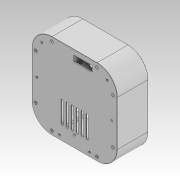
# Autodesk Inventor part: J1_Base
Saved by Autodesk Inventor 2020 (Build 240168000, 168)
## iProperties
Created: 2021-03-23
Part Number: J1_Base
Material: Generic
Document SubType Name: Modeling
Designer: DDeGo
Density: 1 g/cm^3
Appearance: Default
Author: DDeGo
Autodesk Inventor part; units mm, degrees
sketch "Block1" plane through (0, 0, 0) normal (0, 0, 1) x (1, 0, 0)
  circle A0 centre (112.1187, 97.7562) radius 2.75
  line L0 (90.8687, 90.2562) -> (90.8687, 49.9679) construction
  circle A1 centre (83.3687, 50.2562) radius 2.75
  line L1 (75.8687, 49.9679) -> (75.8687, 122.7562) construction
  line L2 (75.8687, 49.9679) -> (90.8687, 49.9679) construction
  circle A2 centre (83.3687, 115.2562) radius 2.75
  line L3 (90.8687, 90.2562) -> (190.8687, 90.2562) construction
  line L4 (75.8687, 122.7562) -> (205.8687, 122.7562) construction
  circle A3 centre (140.8687, 115.2562) radius 2.75
  circle A4 centre (169.6187, 97.7562) radius 2.75
  circle A5 centre (198.3687, 115.2562) radius 2.75
  line L5 (190.8687, 90.2562) -> (190.8687, 40.2562) construction
  line L6 (205.8687, 40.2562) -> (205.8687, 122.7562) construction
  circle A6 centre (198.3687, 50.2562) radius 2.75
  line L7 (205.8687, 40.2562) -> (190.8687, 40.2562) construction
  line L8 (83.3687, 115.2562) -> (140.8687, 115.2562) construction
  line L9 (140.8687, 115.2562) -> (198.3687, 115.2562) construction
  line L10 (198.3687, 115.2562) -> (198.3687, 50.2562) construction
  line L11 (198.3687, 50.2562) -> (83.3687, 50.2562) construction
  line L12 (83.3687, 50.2562) -> (83.3687, 115.2562) construction
  line L13 (112.1187, 115.2562) -> (112.1187, 97.7562) construction
  line L14 (169.6187, 115.2562) -> (169.6187, 97.7562) construction
  line L15 (169.6187, 97.7562) -> (112.1187, 97.7562) construction
  point P0 (142.3997, 87.8737)
  point P1 (140.8687, 90.2562)
  point P2 (140.8687, 90.2562)
  dimension "d9" = 5.5
  dimension "d10" = 57.5
  dimension "d11" = 7.5
  dimension "d12" = 7.5
  dimension "d13" = 7.5
  dimension "d14" = 17.5
  dimension "d15" = 7.5
  dimension "d16" = 10
  dimension "d17" = 65
  dimension "d18" = 7.5
  dimension "d19" = 7.5
  measures "d9" diameter of A0
  measures "d10" distance of L8.start L8.end
  measures "d11" distance between parallel lines of L6 L10
  measures "d12" distance between parallel lines of L4 L9
  measures "d13" distance between parallel lines of L1 L12
  measures "d14" distance of L13.start L13.end
  measures "d15" distance between parallel lines of L3 L15
  measures "d16" distance between parallel lines of L7 L11
  measures "d17" distance of L9.end L10.end
  measures "d18" distance from line of L5 L10.end
  measures "d19" distance between parallel lines of L12 L0
sketch "Sketch1" plane through (0, 0, 0) normal (0, 0, 1) x (1, 0, 0)
  line L0 (45, -85) -> (-45, -85)
  line L1 (-85, -45) -> (-85, 45)
  line L2 (-45, 85) -> (45, 85)
  line L3 (85, 45) -> (85, -45)
  line L4 (85, -85) -> (-85, 85) construction
  line L5 (-85, -85) -> (85, 85) construction
  arc A0 (-45, 85) -> (-85, 45) centre (-45, 45) ccw
  arc A1 (85, 45) -> (45, 85) centre (45, 45) ccw
  arc A2 (45, -85) -> (85, -45) centre (45, -45) ccw
  arc A3 (-85, -45) -> (-45, -85) centre (-45, -45) ccw
  point P0 (0, 0)
  dimension "d1" = 170
  dimension "d2" = 170
  dimension "d3" = 40
  constraints: 12 end point, 8 point on circle, 8 point on line, 8 tangent, 4 centre point, 3 equal radius, 2 midpoint, 2 parallel, 1 horizontal, 1 perpendicular
  measures "d1" distance between parallel lines of L3 L1
  measures "d2" distance between parallel lines of L0 L2
  measures "d3" radius of A0
extrude "Extrusion1" add sketch "Sketch1" along normal blind 62
sketch "Sketch2" plane through (0, 0, 62) normal (0, 0, 1) x (1, 0, 0)
  line L0 (0, 0) -> (-85, 0) construction
  line L1 (-85, 45) -> (-85, -45) projected
  line L2 (0, 0) -> (0, 52.5) construction
  line L3 (45, 85) -> (-45, 85) projected
  circle A0 centre (-28.75, 60) radius 2.75
  line L4 (-50, 52.5) -> (-50, 12.2116) construction
  circle A1 centre (-57.5, 12.5) radius 2.75
  line L5 (-65, 12.2116) -> (-65, 85) construction
  line L6 (-65, 12.2116) -> (-50, 12.2116) construction
  circle A2 centre (-57.5, 77.5) radius 2.75
  line L7 (-50, 52.5) -> (50, 52.5) construction
  line L8 (-65, 85) -> (65, 85) construction
  circle A3 centre (0, 77.5) radius 2.75
  circle A4 centre (28.75, 60) radius 2.75
  circle A5 centre (57.5, 77.5) radius 2.75
  line L9 (50, 52.5) -> (50, 2.5) construction
  line L10 (65, 2.5) -> (65, 85) construction
  circle A6 centre (57.5, 12.5) radius 2.75
  line L11 (65, 2.5) -> (50, 2.5) construction
  line L12 (-57.5, 77.5) -> (0, 77.5) construction
  line L13 (0, 77.5) -> (57.5, 77.5) construction
  line L14 (57.5, 77.5) -> (57.5, 12.5) construction
  line L15 (57.5, 12.5) -> (-57.5, 12.5) construction
  line L16 (-57.5, 12.5) -> (-57.5, 77.5) construction
  line L17 (-28.75, 77.5) -> (-28.75, 60) construction
  line L18 (28.75, 77.5) -> (28.75, 60) construction
  line L19 (28.75, 60) -> (-28.75, 60) construction
  circle A7 centre (-28.75, -60) radius 2.75
  line L20 (-50, -52.5) -> (-50, -12.2116) construction
  circle A8 centre (-57.5, -12.5) radius 2.75
  line L21 (-65, -12.2116) -> (-65, -85) construction
  line L22 (-65, -12.2116) -> (-50, -12.2116) construction
  circle A9 centre (-57.5, -77.5) radius 2.75
  line L23 (-50, -52.5) -> (50, -52.5) construction
  line L24 (-65, -85) -> (65, -85) construction
  circle A10 centre (0, -77.5) radius 2.75
  circle A11 centre (28.75, -60) radius 2.75
  circle A12 centre (57.5, -77.5) radius 2.75
  line L25 (50, -52.5) -> (50, -2.5) construction
  line L26 (65, -2.5) -> (65, -85) construction
  circle A13 centre (57.5, -12.5) radius 2.75
  line L27 (65, -2.5) -> (50, -2.5) construction
  line L28 (-57.5, -77.5) -> (0, -77.5) construction
  line L29 (0, -77.5) -> (57.5, -77.5) construction
  line L30 (57.5, -77.5) -> (57.5, -12.5) construction
  line L31 (57.5, -12.5) -> (-57.5, -12.5) construction
  line L32 (-57.5, -12.5) -> (-57.5, -77.5) construction
  line L33 (-28.75, -77.5) -> (-28.75, -60) construction
  line L34 (28.75, -77.5) -> (28.75, -60) construction
  line L35 (28.75, -60) -> (-28.75, -60) construction
  constraints: 4 end point, 2 horizontal, 1 midpoint, 1 vertical, 2 other
extrude "Extrusion2" [suppressed]
ref_plane "Work Plane1" through (0, 0, -15) normal (0, 0, -1) x (-1, 0, 0)
sketch "Sketch3" plane through (0, 0, -15) normal (0, 0, -1) x (-1, 0, 0)
  circle A0 centre (0, 0) radius 87.5
  line L0 (-85, -45) -> (-85, 45) construction
  dimension "d27" = 175
  constraints: 1 centre point, 1 coincident
  measures "d27" diameter of A0
sketch "Sketch4" plane through (0, 0, 0) normal (0, 0, -1) x (-1, 0, 0)
  line L0 (-85, -45) -> (-85, 45) projected
  arc A0 (-85, -45) -> (-45, -85) centre (-45, -45) ccw projected
  line L1 (45, -85) -> (-45, -85) projected
  arc A1 (45, -85) -> (85, -45) centre (45, -45) ccw projected
  line L2 (85, 45) -> (85, -45) projected
  arc A2 (85, 45) -> (45, 85) centre (45, 45) ccw projected
  line L3 (-45, 85) -> (45, 85) projected
  arc A3 (-45, 85) -> (-85, 45) centre (-45, 45) ccw projected
  point P0 (0, 0)
loft "Loft1" add profiles "Sketch3", "Sketch4"
sketch "Sketch5" plane through (0, 0, -15) normal (0, 0, -1) x (-1, 0, 0)
  arc A0 (-37.1204, 79.2359) -> (-77.3314, 40.9402) centre (0, 0) ccw projected
  arc A1 (-77.3314, 40.9402) -> (-77.3314, -40.9402) centre (0, 0) ccw projected
  arc A2 (-77.3314, -40.9402) -> (-40.9402, -77.3314) centre (0, 0) ccw projected
  arc A3 (-40.9402, -77.3314) -> (40.9402, -77.3314) centre (0, 0) ccw projected
  arc A4 (40.9402, -77.3314) -> (77.3314, -40.9402) centre (0, 0) ccw projected
  arc A5 (77.3314, -40.9402) -> (77.3314, 40.9402) centre (0, 0) ccw projected
  arc A6 (77.3314, 40.9402) -> (40.9402, 77.3314) centre (0, 0) ccw projected
  arc A7 (40.9402, 77.3314) -> (-37.1204, 79.2359) centre (0, 0) ccw projected
extrude "Extrusion3" add sketch "Sketch5" along normal blind 5
ref_plane "Work Plane2" through (0, 0, 60.5) normal (0, 0, 1) x (1, 0, 0)
sketch "Sketch6" plane through (0, 0, 60.5) normal (0, 0, 1) x (1, 0, 0)
  arc A0 (-45, 85) -> (-85, 45) centre (-45, 45) ccw projected
  line L0 (-85, 45) -> (-85, -45) projected
  arc A1 (-85, -45) -> (-45, -85) centre (-45, -45) ccw projected
  line L1 (-45, -85) -> (45, -85) projected
  arc A2 (45, -85) -> (85, -45) centre (45, -45) ccw projected
  line L2 (85, -45) -> (85, 45) projected
  arc A3 (85, 45) -> (45, 85) centre (45, 45) ccw projected
  line L3 (45, 85) -> (-45, 85) projected
  line L4 (-82.5, -45) -> (-82.5, 45)
  arc A4 (-45, 82.5) -> (-82.5, 45) centre (-45, 45) ccw
  line L5 (-45, 82.5) -> (45, 82.5)
  arc A5 (82.5, 45) -> (45, 82.5) centre (45, 45) ccw
  line L6 (82.5, 45) -> (82.5, -45)
  arc A6 (45, -82.5) -> (82.5, -45) centre (45, -45) ccw
  line L7 (45, -82.5) -> (-45, -82.5)
  arc A7 (-82.5, -45) -> (-45, -82.5) centre (-45, -45) ccw
  line L8 (-85, 45) -> (-85, -45) projected
  point P0 (0, 0)
  dimension "d29" = 2.5
  constraints: 8 end point, 8 point on circle, 4 centre point, 7 other
  measures "d29" distance between parallel lines of L8 L4
ref_plane "Work Plane3" through (85, -45, 0) normal (0, 0, -1) x (-1, 0, 0)
sketch "Sketch7" plane through (85, -45, 0) normal (0, 0, -1) x (-1, 0, 0)
  arc A0 (170, 90) -> (130, 130) centre (130, 90) ccw projected
  line L0 (170, 90) -> (170, 0) projected
  arc A1 (130, -40) -> (170, 0) centre (130, 0) ccw projected
  line L1 (130, -40) -> (40, -40) projected
  arc A2 (0, 0) -> (40, -40) centre (40, 0) ccw projected
  line L2 (0, 0) -> (0, 90) projected
  arc A3 (40, 130) -> (0, 90) centre (40, 90) ccw projected
  line L3 (40, 130) -> (130, 130) projected
  line L4 (166, 0) -> (166, 90)
  arc A4 (166, 90) -> (130, 126) centre (130, 90) ccw
  line L5 (130, 126) -> (40, 126)
  arc A5 (40, 126) -> (4, 90) centre (40, 90) ccw
  line L6 (4, 90) -> (4, 0)
  arc A6 (4, 0) -> (40, -36) centre (40, 0) ccw
  line L7 (40, -36) -> (130, -36)
  arc A7 (130, -36) -> (166, 0) centre (130, 0) ccw
  point P0 (85, 45)
  dimension "d30" = 4
  constraints: 8 end point, 8 point on circle, 4 centre point, 7 other
  measures "d30" distance between parallel lines of L0 L4
extrude "Extrusion4" cut sketch "Sketch6" against normal up to surface (60.5 mm away) contours L4 A4 L5 A5 L6 A6 L7 A7
sketch "Sketch8" plane through (0, 0, -20) normal (0, 0, -1) x (-1, 0, 0)
  circle A0 centre (0, 0) radius 72.5
  dimension "d33" = 145
  constraints: 1 centre point, 1 coincident
  measures "d33" diameter of A0
extrude "Extrusion5" cut sketch "Sketch8" against normal blind 29.75
sketch "Sketch10" plane through (0, 0, 60.5) normal (0, 0, -1) x (-1, 0, 0)
  line L0 (1, 64) -> (-35, 64)
  line L1 (-35, 64) -> (-35, 75.4)
  line L2 (-35, 75.4) -> (1, 75.4)
  line L3 (1, 75.4) -> (1, 64)
  line L4 (-45, 85) -> (45, 85) projected
  point P0 (0, 0)
  point P1 (0, 85)
  dimension "d69" = 9.6
  dimension "d70" = 21
  dimension "d71" = 1
  dimension "d72" = 35
  constraints: 8 end point, 2 parallel, 1 horizontal, 1 midpoint, 1 perpendicular
  measures "d69" distance between parallel lines of L4 L2
  measures "d70" distance between parallel lines of L4 L0
  measures "d71" distance from line of L3 point (0, 85)
  measures "d72" distance from line of L1 point (0, 85)
extrude "Extrusion7" cut sketch "Sketch10" against normal through all
sketch "Sketch11" plane through (0, 0, 62) normal (0, 0, 1) x (1, 0, 0)
  line L0 (-24.2935, -55) -> (-24.2935, -15) construction
  line L1 (-26.7935, -55) -> (-26.7935, -15)
  line L2 (-21.7935, -15) -> (-21.7935, -55)
  arc A0 (-26.7935, -55) -> (-21.7935, -55) centre (-24.2935, -55) ccw
  arc A1 (-21.7935, -15) -> (-26.7935, -15) centre (-24.2935, -15) ccw
  line L3 (0, 0) -> (68.8945, 0) construction
  line L4 (-14.2935, -55) -> (-14.2935, -15) construction
  line L5 (-16.7935, -55) -> (-16.7935, -15)
  line L6 (-11.7935, -15) -> (-11.7935, -55)
  arc A2 (-16.7935, -55) -> (-11.7935, -55) centre (-14.2935, -55) ccw
  arc A3 (-11.7935, -15) -> (-16.7935, -15) centre (-14.2935, -15) ccw
  line L7 (-4.2935, -55) -> (-4.2935, -15) construction
  line L8 (-6.7935, -55) -> (-6.7935, -15)
  line L9 (-1.7935, -15) -> (-1.7935, -55)
  arc A4 (-6.7935, -55) -> (-1.7935, -55) centre (-4.2935, -55) ccw
  arc A5 (-1.7935, -15) -> (-6.7935, -15) centre (-4.2935, -15) ccw
  line L10 (5.7065, -55) -> (5.7065, -15) construction
  line L11 (3.2065, -55) -> (3.2065, -15)
  line L12 (8.2065, -15) -> (8.2065, -55)
  arc A6 (3.2065, -55) -> (8.2065, -55) centre (5.7065, -55) ccw
  arc A7 (8.2065, -15) -> (3.2065, -15) centre (5.7065, -15) ccw
  line L13 (15.7065, -55) -> (15.7065, -15) construction
  line L14 (13.2065, -55) -> (13.2065, -15)
  line L15 (18.2065, -15) -> (18.2065, -55)
  arc A8 (13.2065, -55) -> (18.2065, -55) centre (15.7065, -55) ccw
  arc A9 (18.2065, -15) -> (13.2065, -15) centre (15.7065, -15) ccw
  line L16 (25.7065, -55) -> (25.7065, -15) construction
  line L17 (23.2065, -55) -> (23.2065, -15)
  line L18 (28.2065, -15) -> (28.2065, -55)
  arc A10 (23.2065, -55) -> (28.2065, -55) centre (25.7065, -55) ccw
  arc A11 (28.2065, -15) -> (23.2065, -15) centre (25.7065, -15) ccw
  point P0 (-24.2935, -35)
  point P1 (-14.2935, -35)
  point P2 (-4.2935, -35)
  point P3 (5.7065, -35)
  point P4 (15.7065, -35)
  point P5 (25.7065, -35)
  dimension "d44" = 2.5
  dimension "d47" = 10
  dimension "d92" = 55
  dimension "d93" = 15
  constraints: 50 end point, 24 point on circle, 12 centre point, 4 tangent, 2 horizontal, 1 midpoint, 1 parallel, 1 vertical, 60 other
  measures "d44" radius of A1
  measures "d47" distance of L1.start L5.start
  measures "d92" distance from line of L13.start L3
  measures "d93" distance from line of L13.end L3
extrude "Extrusion8" cut sketch "Sketch11" against normal blind 10
sketch "Sketch12" plane through (-45, 82.5, 0) normal (0, 0, 1) x (1, 0, 0)
  circle A0 centre (38.7385, -72.8833) radius 193.3593
  point P0 (45, -82.5)
  constraints: 1 centre point
extrude "SnipSnip" cut sketch "Sketch12" against normal through all
sketch "Sketch13" plane through (-45, -85, 62) normal (0, -1, 0) x (1, 0, 0)
  line L0 (7.3311, -8.6737) -> (24.3174, -8.6737)
  line L1 (24.3174, -8.6737) -> (24.3174, -15.7888)
  line L2 (24.3174, -15.7888) -> (7.3311, -15.7888)
  line L3 (7.3311, -15.7888) -> (7.3311, -8.6737)
  line L4 (61.8635, -8.6737) -> (77.0118, -8.6737)
  line L5 (77.0118, -8.6737) -> (77.0118, -15.7888)
  line L6 (77.0118, -15.7888) -> (61.8635, -15.7888)
  line L7 (61.8635, -15.7888) -> (61.8635, -8.6737)
  point P0 (45, -62)
  constraints: 16 end point, 4 parallel, 2 horizontal, 2 perpendicular, 1 point on line
extrude "Extrusion10" cut sketch "Sketch13" against normal blind 10
sketch "Sketch14" plane through (-45, 82.5, 0) normal (0, 0, -1) x (-1, 0, 0)
  arc A0 (0, -165) -> (37.5, -127.5) centre (0, -127.5) ccw projected
  line L0 (0, -165) -> (-90, -165) projected
  arc A1 (-127.5, -127.5) -> (-90, -165) centre (-90, -127.5) ccw projected
  line L1 (-127.5, -127.5) -> (-127.5, -37.5) projected
  arc A2 (-90, 0) -> (-127.5, -37.5) centre (-90, -37.5) ccw projected
  line L2 (-90, 0) -> (0, 0) projected
  arc A3 (37.5, -37.5) -> (0, 0) centre (0, -37.5) ccw projected
  line L3 (37.5, -37.5) -> (37.5, -127.5) projected
  arc A4 (-90, 2.5) -> (-130, -37.5) centre (-90, -37.5) ccw projected
  line L4 (-130, -127.5) -> (-130, -37.5) projected
  arc A5 (-130, -127.5) -> (-90, -167.5) centre (-90, -127.5) ccw projected
  line L5 (0, -167.5) -> (-90, -167.5) projected
  arc A6 (0, -167.5) -> (40, -127.5) centre (0, -127.5) ccw projected
  line L6 (40, -37.5) -> (40, -127.5) projected
  arc A7 (40, -37.5) -> (0, 2.5) centre (0, -37.5) ccw projected
  line L7 (-90, 2.5) -> (0, 2.5) projected
  line L8 (-90, -37.5) -> (-90, -5.5) construction
  line L9 (-90, -37.5) -> (-122, -37.5) construction
  line L10 (-90, -37.5) -> (-45, -82.5) construction
  circle A8 centre (-122, -37.5) radius 2.75
  circle A9 centre (-90, -5.5) radius 2.75
  arc A10 (-93.75, -5.5) -> (-86.25, -5.5) centre (-90, -5.5) ccw
  line L11 (-90, 0) -> (0, 0) projected
  arc A11 (-122, -41.25) -> (-122, -33.75) centre (-122, -37.5) ccw
  line L12 (-127.5, -127.5) -> (-127.5, -37.5) projected
  line L13 (-122, -41.25) -> (-127.5, -41.25)
  line L14 (-122, -33.75) -> (-127.5, -33.75)
  line L15 (-93.75, -5.5) -> (-93.75, 0)
  line L16 (-86.25, -5.5) -> (-86.25, 0)
  line L17 (-86.25, -159.5) -> (-86.25, -165)
  arc A12 (-86.25, -159.5) -> (-93.75, -159.5) centre (-90, -159.5) ccw
  line L18 (-93.75, -159.5) -> (-93.75, -165)
  circle A13 centre (-90, -159.5) radius 2.75
  line L19 (-122, -123.75) -> (-127.5, -123.75)
  arc A14 (-122, -131.25) -> (-122, -123.75) centre (-122, -127.5) ccw
  circle A15 centre (-122, -127.5) radius 2.75
  line L20 (-122, -131.25) -> (-127.5, -131.25)
  line L21 (32, -123.75) -> (37.5, -123.75)
  arc A16 (32, -123.75) -> (32, -131.25) centre (32, -127.5) ccw
  line L22 (32, -131.25) -> (37.5, -131.25)
  circle A17 centre (32, -127.5) radius 2.75
  line L23 (-3.75, -159.5) -> (-3.75, -165)
  arc A18 (3.75, -159.5) -> (-3.75, -159.5) centre (0, -159.5) ccw
  circle A19 centre (0, -159.5) radius 2.75
  line L24 (3.75, -159.5) -> (3.75, -165)
  line L25 (-3.75, -5.5) -> (-3.75, 0)
  arc A20 (-3.75, -5.5) -> (3.75, -5.5) centre (0, -5.5) ccw
  line L26 (3.75, -5.5) -> (3.75, 0)
  circle A21 centre (0, -5.5) radius 2.75
  line L27 (32, -41.25) -> (37.5, -41.25)
  arc A22 (32, -33.75) -> (32, -41.25) centre (32, -37.5) ccw
  circle A23 centre (32, -37.5) radius 2.75
  line L28 (32, -33.75) -> (37.5, -33.75)
  point P0 (-90, -165)
  point P1 (-90, -167.5)
  point P2 (-127.5, -127.5)
  point P3 (-130, -127.5)
  point P4 (37.5, -127.5)
  point P5 (40, -127.5)
  point P6 (0, -165)
  point P7 (0, -167.5)
  point P8 (0, 0)
  point P9 (0, 2.5)
  point P10 (37.5, -37.5)
  point P11 (37.5, -41.25)
  point P12 (37.312, -33.75)
  point P13 (37.312, -131.25)
  point P14 (37.5, -123.75)
  point P15 (-127.312, -131.25)
  point P16 (-127.312, -33.75)
  point P17 (-127.5, -41.25)
  point P18 (-93.75, -0.188)
  point P19 (3.75, -0.188)
  point P20 (-3.75, 0)
  point P21 (-3.75, -165)
  point P22 (3.75, -164.812)
  point P23 (-93.75, -164.812)
  point P24 (-86.25, -165)
  dimension "d59" = 45
  dimension "d60" = 5.5
  dimension "d63" = 360
  dimension "d73" = 8
  dimension "d126" = 32
  dimension "d149" = 1
  dimension "d150" = 1
  constraints: 38 end point, 16 centre point, 16 coincident, 16 point on circle, 5 perpendicular, 4 point on line, 4 tangent, 1 equal radius, 106 other
  measures "d59" angle of L10 L8
  measures "d60" diameter of A9
  measures "d73" distance from line of L7 L8.end
  measures "d126" distance of L8.start L8.end
  measures "d149" radial gap between concentric circles of A10 A9
  measures "d150" radial gap between concentric circles of A11 A8
extrude "Extrusion11" add sketch "Sketch14" against normal up to surface (60.5 mm away) contours L0 L23 A18 L24 A0 | L22 A16 L21 L3 A0 | L0 A1 L18 A12 L17 | L27 A22 L28 A3 L3 | A1 L1 L19 A14 L20 | L26 A20 L25 L2 A3 | L1 A2 L14 A11 L13 | L16 A10 L15 A2 L2
sketch "Sketch15" plane through (-45, 82.5, 0) normal (0, 0, -1) x (-1, 0, 0)
  circle A0 centre (-122, -37.5) radius 2.75 projected
  circle A1 centre (-122, -127.5) radius 2.75 projected
  circle A2 centre (32, -127.5) radius 2.75 projected
  circle A3 centre (32, -37.5) radius 2.75 projected
  circle A4 centre (-90, -159.5) radius 2.75 projected
  circle A5 centre (0, -159.5) radius 2.75 projected
  circle A6 centre (-90, -5.5) radius 2.75 projected
  circle A7 centre (0, -5.5) radius 2.75 projected
  point P0 (-45, -82.5)
extrude "Extrusion12" cut sketch "Sketch15" against normal through all
sketch "Sketch18" plane through (0, 0, 60.5) normal (0, 0, -1) x (-1, 0, 0)
  line L0 (-37.05, -19) -> (37.05, -19) construction
  line L1 (37.05, -19) -> (37.05, -71) construction
  line L2 (37.05, -71) -> (-37.05, -71) construction
  line L3 (-37.05, -71) -> (-37.05, -19) construction
  line L4 (-37.05, -19) -> (37.05, -71) construction
  line L5 (37.05, -19) -> (-37.05, -71) construction
  circle A0 centre (37.05, -19) radius 1.2
  circle A1 centre (37.05, -71) radius 1.2
  circle A2 centre (-37.05, -71) radius 1.2
  circle A3 centre (-37.05, -19) radius 1.2
  line L6 (0, 0) -> (0, -45) construction
  line L7 (-18.2065, -55) -> (-18.2065, -15) construction
  circle A4 centre (37.05, -19) radius 3
  circle A5 centre (37.05, -71) radius 3
  circle A6 centre (-37.05, -71) radius 3
  circle A7 centre (-37.05, -19) radius 3
  line L8 (0, -45) -> (0, -45) construction
  dimension "d94" = 74.1
  dimension "d95" = 52
  dimension "d96" = 2.4
  dimension "d97" = 45
  dimension "d99" = 6
  dimension "d145" = 0
  constraints: 16 end point, 8 centre point, 8 coincident, 6 equal radius, 3 parallel, 2 horizontal, 1 midpoint, 1 perpendicular
  measures "d94" distance of L1.end L2.end
  measures "d95" distance of L0.end L1.end
  measures "d96" diameter of A1
  measures "d97" distance of L6.start L6.end
  measures "d99" diameter of A4
  measures "d145" distance of L6.end L8.end
extrude "Extrusion14" add sketch "Sketch18" along normal blind 7
ref_plane "Work Plane4" through (-41.25, 56.5, 60.5) normal (0, -1, 0) x (1, 0, 0)
sketch "Sketch19" plane through (-41.25, 56.5, 60.5) normal (0, -1, 0) x (1, 0, 0)
  line L0 (97.75, -56.2) -> (40.75, -56.2)
  line L1 (40.75, -56.2) -> (40.75, 0)
  line L2 (40.75, 0) -> (97.75, 0)
  line L3 (97.75, 0) -> (97.75, -56.2)
  line L4 (97.75, -56.2) -> (40.75, 0) construction
  line L5 (40.75, -56.2) -> (97.75, 0) construction
  line L6 (92.75, -4.6) -> (45.75, -4.6) construction
  line L7 (45.75, -4.6) -> (45.75, -51.6) construction
  line L8 (45.75, -51.6) -> (92.75, -51.6) construction
  line L9 (92.75, -51.6) -> (92.75, -4.6) construction
  line L10 (92.75, -4.6) -> (45.75, -51.6) construction
  line L11 (45.75, -4.6) -> (92.75, -51.6) construction
  line L12 (82.5, 0) -> (0, 0) construction
  circle A0 centre (92.75, -51.6) radius 2.25
  circle A1 centre (45.75, -51.6) radius 2.25
  circle A2 centre (45.75, -4.6) radius 2.25
  circle A3 centre (92.75, -4.6) radius 2.25
  circle A4 centre (69.25, -28.1) radius 20
  point P0 (41.25, -60.5)
  point P1 (69.25, -28.1)
  point P2 (41.25, 0)
  dimension "d103" = 57
  dimension "d104" = 47
  dimension "d105" = 28
  dimension "d106" = 4.5
  dimension "d107" = 40
  dimension "d110" = 56.2
  constraints: 24 end point, 6 midpoint, 5 centre point, 5 coincident, 4 parallel, 3 equal radius, 3 perpendicular, 2 horizontal, 1 collinear
  measures "d103" distance of L0.start L0.end
  measures "d104" distance of L7.end L8.end
  measures "d105" horizontal distance of point (69.25, -28.1) point (41.25, 0)
  measures "d106" diameter of A0
  measures "d107" diameter of A4
  measures "d110" distance of L2.end L0.start
extrude "Extrusion15" add sketch "Sketch19" against normal blind 5
sketch "Sketch20" plane through (56.5, 56.5, 60.5) normal (1, 0, 0) x (0, 0, -1)
  line L0 (56.2, 0) -> (0, 0) construction
  line L1 (56.2, 0) -> (56.2, 5) projected
  line L2 (0, 5) -> (56.2, 5) projected
  line L3 (0, 0) -> (0, 5) projected
  line L4 (56.2, 0) -> (0, -32.4471)
  line L5 (0, 0) -> (0, 5) projected
  line L6 (0, -32.4471) -> (0, 0)
  point P0 (60.5, -56.5)
  dimension "d111" = 60
  constraints: 4 end point, 1 collinear
  measures "d111" angle of L6 L4
extrude "Extrusion16" add sketch "Sketch20" along normal blind 3
sketch "Sketch21" plane through (0, 0, 60.5) normal (0, 0, -1) x (-1, 0, 0)
  line L0 (0.5, 61.5) -> (0.5, 56.5) projected
  line L1 (-41.25, 82.5) -> (41.25, 82.5) projected
  line L2 (0.5, 56.5) -> (3.5, 56.5)
  line L3 (3.5, 56.5) -> (3.5, 82.5)
  line L4 (3.5, 82.5) -> (0.5, 82.5)
  line L5 (0.5, 82.5) -> (0.5, 56.5)
  line L6 (-59.5, 61.5) -> (0.5, 61.5) projected
  line L7 (-59.5, 61.5) -> (-56.5, 61.5)
  line L8 (-56.5, 61.5) -> (-56.5, 82.5)
  line L9 (-56.5, 82.5) -> (-59.5, 82.5)
  line L10 (-59.5, 82.5) -> (-59.5, 61.5)
  line L11 (-56.5, 56.5) -> (-56.5, 24.0529) construction
  arc A0 (-48.75, 82.312) -> (-82.312, 48.75) centre (-45, 45) ccw projected
  point P0 (0, 0)
  point P1 (0.5, 82.5)
  point P2 (0.5, 61.5)
  point P3 (-56.5, 80.6931)
  point P4 (-59.5, 79.5832)
  constraints: 16 end point, 5 parallel, 2 horizontal, 2 perpendicular, 2 point on line, 1 collinear
extrude "Extrusion17" add sketch "Sketch21" along normal up to surface (56.2 mm away) contours L5 L1 L3 L2 L0 | L10 A0 L8 L6
sketch "Sketch22" plane through (0, 0, 60.5) normal (0, 0, -1) x (-1, 0, 0)
  circle A0 centre (-75, 0) radius 1.9
  circle A1 centre (-65.0538, 65.0538) radius 1.9
  circle A2 centre (-30, -77) radius 1.9
  circle A3 centre (-45, -77) radius 2.75 construction
  line L0 (-45, -77) -> (-30, -77) construction
  line L1 (-45, 77) -> (-65.0538, 65.0538) construction
  circle A4 centre (-77, 45) radius 2.75 construction
  line L2 (-65.0538, 65.0538) -> (-77, 45) construction
  line L3 (-75, 0) -> (0, 0) construction
  line L4 (0, 0) -> (0, 91.1755) construction
  circle A5 centre (75, 0) radius 1.9
  circle A6 centre (65.0538, 65.0538) radius 1.9
  circle A7 centre (30, -77) radius 1.9
  line L5 (-30, -77) -> (30, -77) construction
  line L6 (0, -77) -> (0, -62) construction
  circle A8 centre (0, -62) radius 1.9
  circle A9 centre (-45, 77) radius 2.75 construction
  dimension "d116" = 75
  dimension "d117" = 92
  dimension "d118" = 3.8
  dimension "d119" = 15
  dimension "d122" = 15
  constraints: 14 end point, 7 centre point, 3 equal radius, 3 horizontal, 3 symmetric about line, 2 coincident, 1 equal length, 1 midpoint, 1 perpendicular, 1 vertical, 3 other
  measures "d116" distance of L3.end L3.start
  measures "d117" distance of L1.end L3.end
  measures "d118" diameter of A0
  measures "d119" distance of L0.start L0.end
  measures "d122" distance of L6.start L6.end
extrude "Extrusion18" cut sketch "Sketch22" against normal through all
sketch "Sketch23" plane through (-41.25, 61.5, 60.5) normal (0, 1, 0) x (1, 0, 0)
  circle A0 centre (45.75, 4.6) radius 2.25 projected
  line L0 (45.75, 8.7569) -> (49.35, 6.6785)
  line L1 (49.35, 6.6785) -> (49.35, 2.5215)
  line L2 (49.35, 2.5215) -> (45.75, 0.4431)
  line L3 (45.75, 0.4431) -> (42.15, 2.5215)
  line L4 (42.15, 2.5215) -> (42.15, 6.6785)
  line L5 (42.15, 6.6785) -> (45.75, 8.7569)
  circle A1 centre (92.75, 51.6) radius 2.25 projected
  line L6 (92.75, 55.7569) -> (96.35, 53.6785)
  line L7 (96.35, 53.6785) -> (96.35, 49.5215)
  line L8 (96.35, 49.5215) -> (92.75, 47.4431)
  line L9 (92.75, 47.4431) -> (89.15, 49.5215)
  line L10 (89.15, 49.5215) -> (89.15, 53.6785)
  line L11 (89.15, 53.6785) -> (92.75, 55.7569)
  circle A2 centre (92.75, 4.6) radius 2.25 projected
  line L12 (92.75, 8.7569) -> (96.35, 6.6785)
  line L13 (96.35, 6.6785) -> (96.35, 2.5215)
  line L14 (96.35, 2.5215) -> (92.75, 0.4431)
  line L15 (92.75, 0.4431) -> (89.15, 2.5215)
  line L16 (89.15, 2.5215) -> (89.15, 6.6785)
  line L17 (89.15, 6.6785) -> (92.75, 8.7569)
  circle A3 centre (45.75, 51.6) radius 2.25 projected
  line L18 (45.75, 47.4431) -> (42.15, 49.5215)
  line L19 (42.15, 49.5215) -> (42.15, 53.6785)
  line L20 (42.15, 53.6785) -> (45.75, 55.7569)
  line L21 (45.75, 55.7569) -> (49.35, 53.6785)
  line L22 (49.35, 53.6785) -> (49.35, 49.5215)
  line L23 (49.35, 49.5215) -> (45.75, 47.4431)
  dimension "d123" = 7.2
  constraints: 48 end point, 4 coincident, 4 vertical, 3 equal length, 52 other
  measures "d123" distance between parallel lines of L19 L22
extrude "Extrusion19" cut sketch "Sketch23" against normal blind 2.5 contours A0 | L0 L1 L2 L3 L4 L5 | A1 | L6 L7 L8 L9 L10 L11 | A2 | L12 L13 L14 L15 L16 L17 | A3 | L18 L19 L20 L21 L22 L23
sketch "Sketch24" plane through (-45, -85, 62) normal (0, -1, 0) x (1, 0, 0)
  line L0 (61.8635, -8.6737) -> (77.0118, -8.6737) projected
  line L1 (77.0118, -8.6737) -> (77.0118, -15.7888) projected
  line L2 (77.0118, -15.7888) -> (61.8635, -15.7888) projected
  line L3 (61.8635, -15.7888) -> (61.8635, -8.6737) projected
  line L4 (7.3311, -8.6737) -> (24.3174, -8.6737) projected
  line L5 (24.3174, -8.6737) -> (24.3174, -15.7888) projected
  line L6 (24.3174, -15.7888) -> (7.3311, -15.7888) projected
  line L7 (7.3311, -15.7888) -> (7.3311, -8.6737) projected
  line L8 (0, -62) -> (90, -62) projected
  line L9 (90, -62) -> (90, 0) projected
  line L10 (0, 0) -> (90, 0) projected
  line L11 (0, -62) -> (0, 0) projected
  point P0 (45, -62)
extrude "Extrusion20" add sketch "Sketch24" against normal up to surface (2.5 mm away) contours L0 L1 L2 L3 | L4 L5 L6 L7
sketch "Sketch26" plane through (-45, -85, 62) normal (0, -1, 0) x (1, 0, 0)
  line L0 (36.45, -7.5) -> (49.45, -7.5)
  line L1 (49.45, -7.5) -> (49.45, -21.5)
  line L2 (49.45, -21.5) -> (36.45, -21.5)
  line L3 (36.45, -21.5) -> (36.45, -7.5)
  line L4 (36.45, -7.5) -> (49.45, -21.5) construction
  line L5 (49.45, -7.5) -> (36.45, -21.5) construction
  line L6 (15.95, -10.5) -> (27.95, -10.5)
  line L7 (27.95, -10.5) -> (27.95, -18.5)
  line L8 (27.95, -18.5) -> (15.95, -18.5)
  line L9 (15.95, -18.5) -> (15.95, -10.5)
  line L10 (15.95, -10.5) -> (27.95, -18.5) construction
  line L11 (27.95, -10.5) -> (15.95, -18.5) construction
  line L12 (9.15, -8.5) -> (6.75, -8.5) construction
  point P0 (45, -62)
  point P1 (42.95, -14.5)
  point P2 (21.95, -14.5)
  point P3 (7.95, -8.5)
  dimension "d126" = 32
  dimension "d129" = 35
  dimension "d131" = 14
  dimension "d132" = 13
  dimension "d134" = 12
  dimension "d135" = 8
  dimension "d143" = 1
  dimension "d151" = 14
  dimension "d152" = 2
  constraints: 24 end point, 5 midpoint, 4 parallel, 2 horizontal, 2 perpendicular
  measures "d129" horizontal distance of point (7.95, -8.5) point (42.95, -14.5)
  measures "d131" distance of L2.end L0.start
  measures "d132" distance of L1.end L2.end
  measures "d134" distance of L6.start L6.end
  measures "d135" distance between parallel lines of L6 L8
  measures "d143" distance from line of L0 point (7.95, -8.5)
  measures "d151" horizontal distance of point (21.95, -14.5) point (7.95, -8.5)
  measures "d152" distance from line of point (7.95, -8.5) L6
extrude "Extrusion21" cut sketch "Sketch26" against normal blind 28
chamfer "Chamfer1" distance 0.5 angle 45 4 edges at (-35.85, -71, 53.5) (38.25, -71, 53.5) (38.25, -19, 53.5) (-35.85, -19, 53.5)
fillet "Fillet1" radius 5 4 edges at (-34.05, -71, 60.5) (40.05, -71, 60.5) (40.05, -19, 60.5) (-34.05, -19, 60.5)
chamfer "Chamfer2" distance 0.5 angle 45 16 edges at (-85, 0, 62) (-73.2843, -73.2843, 62) (0, -85, 62) (73.2843, -73.2843, 62) (85, 0, 62) (73.2843, 73.2843, 62) (0, 85, 62) (-73.2843, 73.2843, 62) (-85, 0, 0) (-73.2843, -73.2843, 0) (0, -85, 0) (73.2843, -73.2843, 0) (85, 0, 0) (73.2843, 73.2843, 0) (0, 85, 0) (-73.2843, 73.2843, 0)
equation "\"d12\" = d11"
equation "\"d13\" = d11"
equation "\"d15\" = d11"
equation "\"d18\" = d11"
equation "\"d19\" = d11"
body "Solid1"
